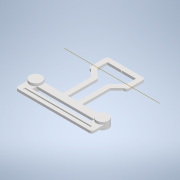
# Autodesk Inventor part: Positioning tool mini VR
Saved by Autodesk Inventor 2021.2 (Build 252289000, 289)
## iProperties
Created: 2021-06-03
Part Number: Positioning tool mini VR
Material: Generic
Document SubType Name: Modeling
Designer: jl4459
Density: 1 g/cm^3
Appearance: Default
Author: jl4459
Autodesk Inventor part; units mm, degrees
ref_plane "YZ Plane" through (0, 0, 0) normal (1, 0, 0) x (0, 1, 0)
ref_plane "XZ Plane" through (0, 0, 0) normal (0, 1, 0) x (-1, 0, 0)
ref_plane "XY Plane" through (0, 0, 0) normal (0, 0, 1) x (1, 0, 0)
sketch "Sketch1" plane through (0, 0, 0) normal (0, 1, 0) x (-1, 0, 0)
  circle A0 centre (88.8958, -0.0003) radius 15.875
  circle A1 centre (-88.8963, -0.0003) radius 15.875
  line L0 (76.1991, 9.5291) -> (-76.1995, 9.5291)
  line L1 (-76.1995, 9.5291) -> (-76.1995, 22.2291)
  line L2 (-76.1995, 22.2291) -> (76.1991, 22.2291)
  line L3 (76.1991, 22.2291) -> (76.1991, 9.5291)
  line L4 (-101.5963, 9.5247) -> (-101.5963, 41.2747)
  line L5 (-101.5963, 41.2747) -> (101.5958, 41.2747)
  line L6 (101.5958, 41.2747) -> (101.5958, 9.5247)
  line L7 (38.1095, -139.6963) -> (-38.0846, -139.6963)
  line L8 (50.8, -152.3702) -> (-50.8, -152.3702)
  line L9 (25.3998, -9.5368) -> (25.3998, -58.2151)
  line L10 (-25.4002, -9.5368) -> (-25.4002, -58.2573)
  line L11 (-25.4002, -9.5368) -> (-76.2049, -9.5368)
  line L12 (-12.6648, -9.5368) -> (12.7095, -9.5368)
  line L13 (25.3998, -9.5368) -> (76.2044, -9.5368)
  line L14 (38.1095, -139.6963) -> (38.1095, -114.2963)
  line L15 (-38.0846, -139.6963) -> (-38.0846, -114.2963)
  line L16 (-50.8, -152.3702) -> (-50.8, -101.5702)
  line L17 (50.8, -152.3702) -> (50.8, -101.5702)
  line L18 (38.1095, -114.2963) -> (12.7095, -88.8963)
  line L19 (38.1095, -114.2963) -> (74.0305, -114.2963) construction
  line L20 (-38.0846, -114.2963) -> (-12.6648, -88.8764)
  line L21 (-38.0846, -114.2963) -> (-2.1355, -114.2963) construction
  line L22 (-12.6648, -9.5368) -> (-12.6648, -88.8764)
  line L23 (12.7095, -9.5368) -> (12.7095, -88.8963)
  line L24 (25.4095, -101.5963) -> (38.1095, -101.5963) construction
  line L25 (38.1095, -114.2963) -> (56.0749, -114.2963) construction
  line L26 (-25.3747, -101.5863) -> (-12.6747, -101.5863) construction
  line L27 (-25.4002, -58.2573) -> (-25.4002, -83.6514)
  line L28 (-50.8, -101.5702) -> (-43.3191, -101.5702)
  line L29 (-43.3191, -101.5702) -> (-25.4002, -83.6514)
  line L30 (25.3998, -58.2151) -> (25.3998, -83.6261)
  line L31 (50.8, -101.5702) -> (43.3439, -101.5702)
  line L32 (25.3998, -83.6261) -> (43.3439, -101.5702)
  point P0 (0, 0)
  dimension "d2" = 31.75
  dimension "d3" = 31.75
  dimension "d119" = 25.4
  dimension "d120" = 25.4
  dimension "d121" = 50.8
  dimension "d122" = 50.8
  dimension "d123" = 135
  dimension "d124" = 45
  constraints: 66 end point, 11 vertical, 10 horizontal, 6 point on circle, 4 perpendicular, 2 centre point, 2 equal length, 2 midpoint, 1 collinear, 1 point on line
  measures "d2" diameter of A0
  measures "d3" diameter of A1
  measures "d119" distance of L7.start L14.end
  measures "d120" distance of L7.end L15.end
  measures "d121" distance of L8.end L16.end
  measures "d122" distance of L8.start L17.end
  measures "d123" angle of L19 L18
  measures "d124" angle of L21 L20
extrude "Extrusion1" add sketch "Sketch1" along normal blind 6.35 contours A0 L3 L2 L1 A1 L4 L5 L6 | L13 L9 L30 L32 L31 L17 L8 L16 L28 L29 L27 L10 L11 A1 L0 A0
sketch "Sketch6" plane through (0, 6.35, 0) normal (0, 1, 0) x (1, 0, 0)
  line L0 (1.2749, 139.6963) -> (-1.2651, 139.6963)
  line L1 (-1.2651, 139.6963) -> (0.0049, 138.4263)
  line L2 (0.0049, 138.4263) -> (1.2749, 139.6963)
  line L3 (38.0856, 115.57) -> (38.0856, 113.03)
  line L4 (38.0856, 113.03) -> (36.8156, 114.3)
  line L5 (36.8156, 114.3) -> (38.0856, 115.57)
  line L6 (-38.1144, 115.57) -> (-38.1144, 113.03)
  line L7 (-38.1144, 113.03) -> (-36.8444, 114.3)
  line L8 (-36.8444, 114.3) -> (-38.1144, 115.57)
  line L9 (12.6648, 9.5368) -> (-12.7095, 9.5368) projected
  line L10 (1.2721, 9.5368) -> (-1.2679, 9.5368)
  line L11 (-1.2679, 9.5368) -> (0.0021, 10.8068)
  line L12 (0.0021, 10.8068) -> (1.2721, 9.5368)
  point P0 (0, 0)
  point P1 (12.6626, 9.5405)
  point P2 (-12.6933, 9.5405)
  point P3 (-12.7095, 9.5368)
  dimension "d55" = 2.54
  dimension "d56" = 45
  dimension "d57" = 2.54
  dimension "d58" = 45
  dimension "d59" = 2.54
  dimension "d60" = 45
  dimension "d61" = 2.54
  dimension "d62" = 45
  constraints: 24 end point, 4 perpendicular, 3 other
  measures "d55" distance of L0.start L0.end
  measures "d56" angle of L1 L0
  measures "d57" distance of L3.start L3.end
  measures "d58" angle of L3 L4
  measures "d59" distance of L6.start L6.end
  measures "d60" angle of L7 L6
  measures "d61" distance of L10.start L10.end
  measures "d62" angle of L10 L11
extrude "Extrusion4" add sketch "Sketch6" against normal blind 6.35
sketch "Sketch13" plane through (0, 6.35, 0) normal (0, 1, 0) x (1, 0, 0)
  circle A0 centre (-88.9, 0) radius 15.875
  circle A1 centre (88.9, 0) radius 15.875
  point P0 (0, 0)
  dimension "d130" = 31.75
  dimension "d131" = 31.75
  constraints: 2 centre point
  measures "d130" diameter of A0
  measures "d131" diameter of A1
extrude "Extrusion5" add sketch "Sketch13" along normal blind 6.35 and the other way blind 12.7
fillet "Fillet1" radius 6.35 10 edges at (101.5963, 3.175, 41.2747) (-101.5958, 3.175, 41.2747) (50.8, 3.175, -152.3702) (-50.8, 3.175, -152.3702) (-50.8, 3.175, -101.5702) (50.8, 3.175, -101.5702) (25.4002, 3.175, -83.6514) (-25.3998, 3.175, -83.6261) (12.6648, 3.175, -88.8764) (-12.7095, 3.175, -88.8963)
sketch "Sketch15" plane through (-88.9, -6.35, 0) normal (0, -1, 0) x (1, 0, 0)
  circle A0 centre (0, 0) radius 15.875 projected
  circle A1 centre (177.8, 0) radius 15.875 projected
  point P0 (88.9, 0)
  constraints: 2 coincident
hole "Hole10" at (-88.9, -6.35, 0) at (88.9, -6.35, 0) direction (0, 1, 0) diameter 26.1938 depth 12.7
sketch "Sketch17" plane through (-88.9, 6.35, 0) normal (0, -1, 0) x (1, 0, 0)
  circle A0 centre (0, 0) radius 13.0969 projected
  circle A1 centre (177.8, 0) radius 13.0969 projected
  point P0 (88.9, 0)
  constraints: 2 coincident
hole "Hole12" at (-88.9, 6.35, 0) at (88.9, 6.35, 0) direction (0, 1, 0) diameter 23.0187 depth 3.175
sketch "Sketch20" plane through (0, 6.35, 0) normal (0, 1, 0) x (1, 0, 0)
  line L0 (-25.3998, 9.5368) -> (-76.2044, 9.5368) projected
  line L1 (-14.5693, 90.7562) -> (-37.4788, 113.6656) projected
  line L2 (76.2049, 9.5368) -> (25.4002, 9.5368) projected
  line L3 (37.452, 113.6636) -> (14.5246, 90.7363) projected
  point P0 (0, 0)
  point P1 (31.7247, 107.9364)
  point P2 (-31.7495, 107.9364)
  dimension "d182" = 98.3996
  dimension "d183" = 0
  dimension "d184" = 98.3996
  dimension "d185" = 0
  measures "d182" distance from line of L0 point (-31.75, 107.936)
  measures "d183" distance from line of L1 point (-31.75, 107.936)
  measures "d184" distance from line of L2 point (31.725, 107.936)
  measures "d185" distance from line of L3 point (31.725, 107.936)
hole "Hole15" at (-31.7495, 6.35, -107.9364) at (31.7247, 6.35, -107.9364) direction (0, -1, 0) diameter 0.7937 end through all
sketch "Sketch21" plane through (0, 6.35, 0) normal (0, 1, 0) x (1, 0, 0)
  line L0 (-25.3998, 9.5368) -> (-76.2044, 9.5368) projected
  line L1 (-14.5693, 90.7562) -> (-31.4689, 107.6557) projected
  line L2 (76.2049, 9.5368) -> (25.4002, 9.5368) projected
  line L3 (31.4441, 107.6557) -> (14.5246, 90.7363) projected
  point P0 (0, 0)
  point P1 (28.5497, 104.7614)
  point P2 (-28.5745, 104.7614)
  dimension "d193" = 95.2246
  dimension "d194" = 0
  dimension "d202" = 95.2246
  dimension "d203" = 0
  measures "d193" distance from line of L0 point (-28.575, 104.761)
  measures "d194" distance from line of L1 point (-28.575, 104.761)
  measures "d202" distance from line of L2 point (28.55, 104.761)
  measures "d203" distance from line of L3 point (28.55, 104.761)
hole "Hole16" at (-28.5745, 6.35, -104.7614) at (28.5497, 6.35, -104.7614) direction (0, -1, 0) diameter 0.7937 end through all
sketch "Sketch22" plane through (0, 6.35, 0) normal (0, 1, 0) x (1, 0, 0)
  line L0 (-25.3998, 9.5368) -> (-76.2044, 9.5368) projected
  line L1 (-14.5693, 90.7562) -> (-28.2939, 104.4807) projected
  line L2 (76.2049, 9.5368) -> (25.4002, 9.5368) projected
  line L3 (28.2691, 104.4807) -> (14.5246, 90.7363) projected
  point P0 (0, 0)
  point P1 (25.3747, 101.5864)
  point P2 (-25.3995, 101.5864)
  dimension "d204" = 92.0496
  dimension "d205" = 0
  dimension "d206" = 92.0496
  dimension "d207" = 0
  measures "d204" distance from line of L0 point (-25.4, 101.586)
  measures "d205" distance from line of L1 point (-25.4, 101.586)
  measures "d206" distance from line of L2 point (25.375, 101.586)
  measures "d207" distance from line of L3 point (25.375, 101.586)
hole "Hole17" at (-25.3995, 6.35, -101.5864) at (25.3747, 6.35, -101.5864) direction (0, -1, 0) diameter 0.7937 end through all
sketch "Sketch23" plane through (0, 6.35, 0) normal (0, 1, 0) x (1, 0, 0)
  line L0 (-25.3998, 9.5368) -> (-76.2044, 9.5368) projected
  line L1 (-14.5693, 90.7562) -> (-25.1189, 101.3057) projected
  line L2 (76.2049, 9.5368) -> (25.4002, 9.5368) projected
  line L3 (25.0941, 101.3057) -> (14.5246, 90.7363) projected
  point P0 (0, 0)
  point P1 (15.8497, 92.0614)
  point P2 (-15.8745, 92.0614)
  dimension "d215" = 82.5246
  dimension "d216" = 0
  dimension "d217" = 82.5246
  dimension "d218" = 0
  measures "d215" distance from line of L0 point (-15.875, 92.061)
  measures "d216" distance from line of L1 point (-15.875, 92.061)
  measures "d217" distance from line of L2 point (15.85, 92.061)
  measures "d218" distance from line of L3 point (15.85, 92.061)
hole "Hole18" at (-15.8745, 6.35, -92.0614) at (15.8497, 6.35, -92.0614) direction (0, -1, 0) diameter 0.7937 end through all
sketch "Sketch25" plane through (0, 6.35, 0) normal (0, 1, 0) x (1, 0, 0)
  line L0 (-88.9, -28.575) -> (88.9, -28.575)
  line L1 (88.9, -28.575) -> (88.9, -34.925)
  line L2 (88.9, -34.925) -> (-88.9, -34.925)
  line L3 (-88.9, -34.925) -> (-88.9, -28.575)
  point P0 (0, 0)
  constraints: 8 end point, 2 parallel, 1 horizontal, 1 perpendicular
extrude "Extrusion7" cut sketch "Sketch25" against normal blind 3.175
body "Solid1"
